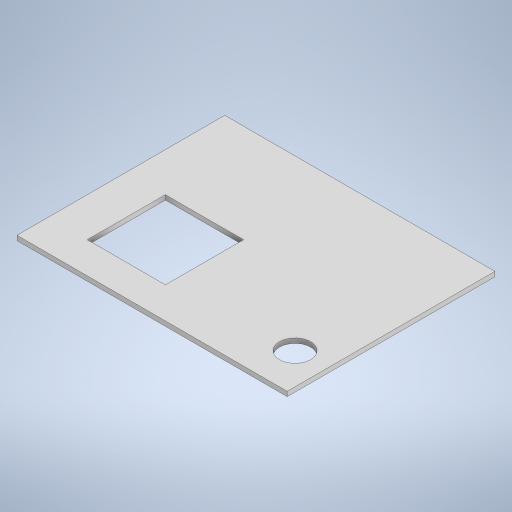
# Autodesk Inventor part: Cabinet - left
Saved by Autodesk Inventor 2024.3 (Build 283343000, 343)
## iProperties
Created: 2025-03-26
Part Number: Cabinet - left
Material: Všeobecné
Document SubType Name: Modeling
Designer: admin
Density: 1 g/cm^3
Appearance: Výchozí
Author: admin
Autodesk Inventor part; units mm, degrees
ref_plane "YZ Plane" through (0, 0, 0) normal (1, 0, 0) x (0, 1, 0)
ref_plane "XZ Plane" through (0, 0, 0) normal (0, 1, 0) x (-1, 0, 0)
ref_plane "XY Plane" through (0, 0, 0) normal (0, 0, 1) x (1, 0, 0)
sketch "Náčrt1" plane through (0, 0, 0) normal (0, 1, 0) x (-1, 0, 0)
  line L0 (0, -93.1) -> (0, 93.1) projected
  line L1 (-121.1, 0) -> (121.1, 0) projected
  line L2 (86.5, 66.5) -> (-86.5, 66.5)
  line L3 (-86.5, 66.5) -> (-86.5, -66.5)
  line L4 (-86.5, -66.5) -> (86.5, -66.5)
  line L5 (86.5, -66.5) -> (86.5, 66.5)
  point P0 (0, 0)
  dimension "d0" = 133
  dimension "d1" = 173
  constraints: 8 end point, 2 parallel, 1 horizontal, 1 perpendicular, 2 other
  measures "d0" distance of L2.end L3.end
  measures "d1" distance of L3.end L4.end
extrude "Vysunutí1" add sketch "Náčrt1" along normal mid plane 3
sketch "Náčrt2" plane through (0, 1.5, 0) normal (0, 1, 0) x (1, 0, 0)
  line L0 (-61.5, -46.5) -> (-11.5, -46.5)
  line L1 (-11.5, -46.5) -> (-11.5, 3.5)
  line L2 (-11.5, 3.5) -> (-61.5, 3.5)
  line L3 (-61.5, 3.5) -> (-61.5, -46.5)
  line L4 (-86.5, -66.5) -> (86.5, -66.5) projected
  line L5 (-86.5, 66.5) -> (-86.5, -66.5) projected
  point P0 (0, 0)
  dimension "d4" = 50
  dimension "d5" = 50
  dimension "d12" = 25
  dimension "d13" = 20
  constraints: 8 end point, 2 parallel, 1 horizontal, 1 perpendicular
  measures "d4" distance of L0.end L1.end
  measures "d5" distance of L1.end L2.end
  measures "d12" distance between parallel lines of L5 L3
  measures "d13" distance between parallel lines of L4 L0
extrude "Vysunutí3" cut sketch "Náčrt2" against normal through all
sketch "Náčrt3" plane through (0, 1.5, 0) normal (0, 1, 0) x (1, 0, 0)
  line L0 (-86.5, -66.5) -> (86.5, -66.5) projected
  line L1 (86.5, -66.5) -> (86.5, 66.5) projected
  point P0 (0, 0)
  point P1 (66.5, -41.5)
  dimension "d19" = 20
  dimension "d20" = 25
  measures "d19" distance from line of L1 point (66.5, -41.5)
  measures "d20" distance from line of L0 point (66.5, -41.5)
hole "Díra1" at (66.5, 1.5, 41.5) direction (0, -1, 0) diameter 20 end through all
